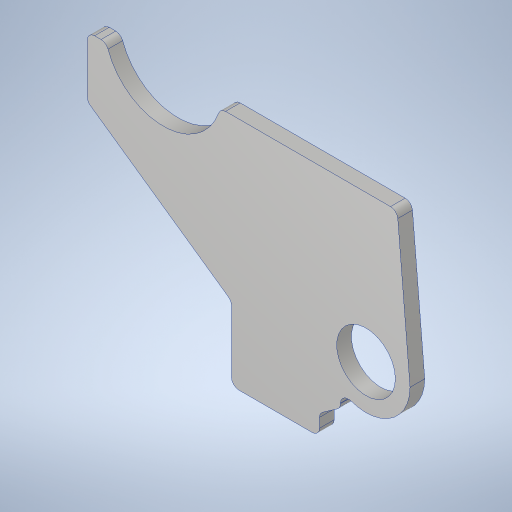
# Autodesk Inventor part: CL1-002
Saved by Autodesk Inventor 2023.4 (Build 274418000, 418)
## iProperties
Created: 2025-01-17
Part Number: CL1-002
Material: Aluminum 6061
Document SubType Name: Modeling
Designer: mavericks
Density: 2.7 g/cm^3
Appearance: Aluminum - Flat
Author: mavericks
Autodesk Inventor part; units mm, degrees
ref_plane "YZ Plane" through (0, 0, 0) normal (1, 0, 0) x (0, 1, 0)
ref_plane "XZ Plane" through (0, 0, 0) normal (0, 1, 0) x (-1, 0, 0)
ref_plane "XY Plane" through (0, 0, 0) normal (0, 0, 1) x (1, 0, 0)
sketch "Sketch1" plane through (0, 0, 0) normal (0, 0, 1) x (1, 0, 0)
  line L0 (-69.85, -50.8) -> (69.85, -50.8) construction
  line L1 (69.85, -50.8) -> (69.85, 50.8) construction
  line L2 (69.85, 50.8) -> (-69.85, 50.8) construction
  line L3 (-69.85, 50.8) -> (-69.85, -50.8) construction
  line L4 (-69.85, -50.8) -> (69.85, 50.8) construction
  line L5 (69.85, -50.8) -> (-69.85, 50.8) construction
  circle A0 centre (-36.9364, 57.15) radius 25.4 construction
  circle A1 centre (50.8, -12.7) radius 12.7 construction
  circle A2 centre (50.8, -12.7) radius 19.05 construction
  line L6 (-69.85, 24.6565) -> (-7.4306, -19.05) construction
  line L7 (-7.4306, -19.05) -> (-7.4306, -50.8) construction
  line L8 (30.6694, -50.8) -> (30.6694, -41.91) construction
  line L9 (30.6694, -41.91) -> (39.7381, -35.56) construction
  line L10 (39.7381, -35.56) -> (39.7381, -30.48) construction
  line L11 (39.7381, -30.48) -> (46.9931, -30.48) construction
  line L12 (46.9931, -30.48) -> (43.9608, -30.48) construction
  line L13 (69.85, -12.7) -> (64.2945, 50.8) construction
  line L14 (-7.4306, -50.8) -> (30.6694, -50.8)
  line L15 (30.6694, -50.8) -> (30.6694, -41.91)
  line L16 (30.6694, -41.91) -> (39.7381, -35.56)
  line L17 (39.7381, -35.56) -> (39.7381, -30.48)
  line L18 (39.7381, -30.48) -> (43.9608, -30.48)
  line L19 (69.85, -12.7) -> (64.2945, 50.8)
  line L20 (64.2945, 50.8) -> (-12.343, 50.8)
  line L21 (-69.85, 50.8) -> (-61.5299, 50.8)
  line L22 (-69.85, 50.8) -> (-69.85, 24.6565)
  line L23 (-69.85, 24.6565) -> (-7.4306, -19.05)
  line L24 (-7.4306, -19.05) -> (-7.4306, -50.8)
  arc A3 (43.9608, -30.48) -> (69.85, -12.7) centre (50.8, -12.7) ccw
  circle A4 centre (50.8, -12.7) radius 12.7
  arc A5 (-61.5299, 50.8) -> (-12.343, 50.8) centre (-36.9364, 57.15) ccw
  point P0 (0, 0)
  dimension "d0" = 101.6
  dimension "d1" = 139.7
  dimension "d3" = 50.8
  dimension "d4" = 6.35
  dimension "d5" = 36.9364
  dimension "d6" = 19.05
  dimension "d7" = 38.1
  dimension "d8" = 38.1
  dimension "d9" = 25.4
  dimension "d10" = 125
  dimension "d11" = 31.75
  dimension "d12" = 76.2
  dimension "d13" = 5.08
  dimension "d14" = 6.35
  dimension "d15" = 8.89
  dimension "d16" = 125
  dimension "d17" = 38.1
  dimension "d18" = 95
  constraints: 50 end point, 9 point on line, 8 collinear, 8 point on circle, 6 centre point, 5 perpendicular, 4 coincident, 3 parallel, 2 midpoint, 1 concentric, 1 horizontal
  measures "d0" distance of L0.end L1.end
  measures "d1" distance of L1.end L2.end
  measures "d3" diameter of A0
  measures "d4" vertical distance of L2.end A0.centre
  measures "d5" horizontal distance of point (0, 0) A0.centre
  measures "d6" distance from line of L1 A1.centre
  measures "d7" distance from line of L0 A1.centre
  measures "d8" diameter of A2
  measures "d9" diameter of A1
  measures "d10" angle of L7 L6
  measures "d11" distance of L6.end L7.end
  measures "d12" distance of L6.start L6.end
  measures "d13" distance of L9.end L10.end
  measures "d14" vertical distance of L8.end L9.end
  measures "d15" distance of L8.start L8.end
  measures "d16" angle of L9 L17
  measures "d17" distance between parallel lines of L15 L7
  measures "d18" angle of L20 L19
extrude "Extrusion1" add sketch "Sketch1" along normal blind 6.35
fillet "Fillet1" radius 3.175 11 edges at (-7.4306, -50.8, 3.175) (30.6694, -50.8, 3.175) (30.6694, -41.91, 3.175) (39.7381, -35.56, 3.175) (39.7381, -30.48, 3.175) (64.2945, 50.8, 3.175) (-12.343, 50.8, 3.175) (-61.5299, 50.8, 3.175) (-69.85, 50.8, 3.175) (-69.85, 24.6565, 3.175) (-7.4306, -19.05, 3.175)
body "Solid1"
